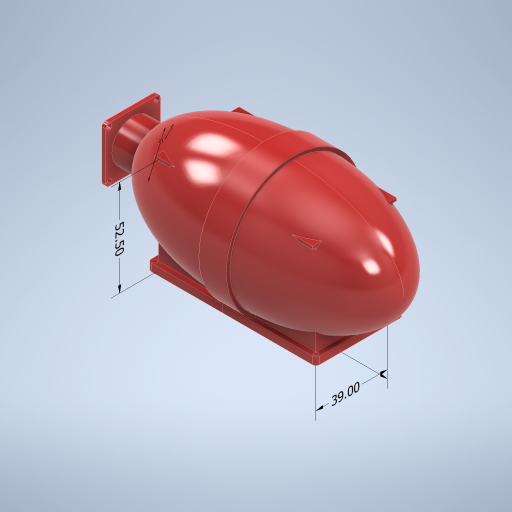
# Autodesk Inventor part: Submarino
Saved by Autodesk Inventor 2023 (Build 270158000, 158)
## iProperties
Created: 2023-03-17
Part Number: Submarino
Material: Plástico PET
Document SubType Name: Modeling
Designer: sergi
Density: 1.541 g/cm^3
Appearance: Rojo naranja
Author: sergi
Autodesk Inventor part; units mm, degrees
note: some values were not read from the file. Chosen so that the rebuilt part matches the saved one: direction of "Agujero2"; direction of "Agujero3"; direction of "Agujero4"; direction of "Agujero5"; direction of "Agujero6"; direction of "Agujero7"; direction of "Agujero8".
ref_plane "XZ Plane" through (0, 0, 0) normal (0, 1, 0) x (-1, 0, 0)
ref_plane "XY Plane" through (0, 0, 0) normal (0, 0, 1) x (1, 0, 0)
sketch "Boceto1" plane through (0, 0, 0) normal (0, 0, 1) x (1, 0, 0)
  line L0 (0, 0) -> (-65, 0)
  line L1 (0, 0) -> (0, 35)
  ellipse E0 centre (0, 0) end of major axis (-65, 0) minor radius 35
  line L2 (0, 0) -> (-63.25, 0)
  line L3 (0, 0) -> (0, 33.25)
  ellipse E1 centre (0, 0) end of major axis (-63.25, 0) minor radius 33.25
  line L4 (0, 0) -> (65, 0)
  point P0 (63.25, 0)
  dimension "d0" = 65
  dimension "d1" = 35
  dimension "d2" = 63.25
  dimension "d3" = 33.25
  constraints: 10 end point, 4 horizontal, 2 coincident, 2 point on line, 1 vertical, 9 other
  measures "d0" distance of L0.start L0.end
  measures "d1" distance of L0.start L1.end
  measures "d2" distance of L2.start L2.end
  measures "d3" distance of L2.start L3.end
revolve "Revolución1" add sketch "Boceto1" angle 360 about axis through (0, 0, 0) along (-1, 0, 0) contours L0 E0 L1 E1 | L1 E0 L4 E1
sketch "Boceto4" plane through (0, 0, 0) normal (0, 1, 0) x (-1, 0, 0)
  line L0 (-36.5, -19.5) -> (36.5, -19.5)
  line L1 (36.5, -19.5) -> (36.5, 19.5)
  line L2 (36.5, 19.5) -> (-36.5, 19.5)
  line L3 (-36.5, 19.5) -> (-36.5, -19.5)
  line L4 (-36.5, -19.5) -> (36.5, 19.5) construction
  line L5 (36.5, -19.5) -> (-36.5, 19.5) construction
  line L6 (-19.5, -14.5) -> (19.5, 14.5) construction
  line L7 (19.5, -14.5) -> (-19.5, 14.5) construction
  line L8 (-38, -21) -> (38, -21)
  line L9 (38, -21) -> (38, 21)
  line L10 (38, 21) -> (-38, 21)
  line L11 (-38, 21) -> (-38, -21)
  line L12 (-38, -21) -> (38, 21) construction
  line L13 (38, -21) -> (-38, 21) construction
  point P0 (0, 0)
  dimension "d21" = 76
  dimension "d22" = 42
  dimension "d44" = 1.5
  dimension "d45" = 1.5
  constraints: 28 end point, 6 midpoint, 4 parallel, 2 horizontal, 2 perpendicular
  measures "d21" distance of L10.end L9.end
  measures "d22" distance of L10.end L8.start
  measures "d44" distance between parallel lines of L10 L2
  measures "d45" distance between parallel lines of L9 L1
extrude "Extrusión1" add sketch "Boceto4" along normal blind 22 and the other way blind 33
extrude "Extrusión2" cut sketch "Boceto4" along normal blind 22 and the other way blind 35 contours L3 L2 L1 L0
sketch "Boceto6" plane through (0, 0, 0) normal (0, 0, 1) x (1, 0, 0)
  point P0 (0, 0)
ref_plane "Plano de trabajo1" through (-60, 0, 0) normal (1, 0, 0) x (0, 1, 0)
sketch "Boceto9" plane through (-60, 0, 0) normal (1, 0, 0) x (0, 1, 0)
  circle A0 centre (0, 0) radius 11.5
  circle A1 centre (0, 0) radius 8.5
  dimension "d46" = 23
  dimension "d49" = 3
  constraints: 2 centre point, 2 coincident
  measures "d46" diameter of A0
  measures "d49" radial gap between concentric circles of A0 A1
extrude "Extrusión5" cut sketch "Boceto9" against normal blind 30 contours A0 | A1
extrude "Extrusión7" cut sketch "Boceto9" along normal blind 10
extrude "Extrusión8" add sketch "Boceto9" along normal mid plane 30
sketch "Boceto10" plane through (-75, 0, 0) normal (-1, 0, 0) x (0, 0, 1)
  line L0 (13, -15) -> (-13, -15)
  line L1 (-15, -13) -> (-15, 13)
  line L2 (-13, 15) -> (13, 15)
  line L3 (15, 13) -> (15, -13)
  line L4 (0, 33.25) -> (0, 0) projected
  line L5 (15, -15) -> (-15, 15) construction
  line L6 (-15, -15) -> (15, 15) construction
  circle A0 centre (0, 0) radius 11.5
  arc A1 (-13, 15) -> (-15, 13) centre (-13, 13) ccw
  arc A2 (-15, -13) -> (-13, -15) centre (-13, -13) ccw
  arc A3 (13, -15) -> (15, -13) centre (13, -13) ccw
  arc A4 (15, 13) -> (13, 15) centre (13, 13) ccw
  point P0 (0, 11.5)
  dimension "d56" = 30
  dimension "d57" = 30
  dimension "d104" = 2
  constraints: 12 end point, 8 point on circle, 8 point on line, 8 tangent, 5 centre point, 3 equal radius, 2 midpoint, 2 parallel, 1 coincident, 1 horizontal, 1 perpendicular
  measures "d56" distance of L5.end L6.end
  measures "d57" distance of L6.start L5.end
  measures "d104" radius of A1
extrude "Extrusión9" add sketch "Boceto10" against normal blind 2
sketch "Boceto12" plane through (0, 22, 0) normal (0, 1, 0) x (1, 0, 0)
  line L0 (-38, 21) -> (38, -21) construction
  line L1 (35, 20) -> (-35, -20) construction
  line L2 (-38, -23) -> (38, -23)
  line L3 (38, -23) -> (38, 23)
  line L4 (38, 23) -> (-38, 23)
  line L5 (-38, 23) -> (-38, -23)
  line L6 (-38, -23) -> (38, 23) construction
  line L7 (38, -23) -> (-38, 23) construction
  point P0 (0, 0)
  dimension "d80" = 76
  dimension "d81" = 46
  constraints: 16 end point, 4 midpoint, 2 parallel, 1 horizontal, 1 perpendicular
  measures "d80" distance of L3.end L4.end
  measures "d81" distance of L4.end L2.start
extrude "Extrusión10" add sketch "Boceto12" against normal blind 1.5
sketch "Boceto14" plane through (0, -33, 0) normal (0, -1, 0) x (1, 0, 0)
  line L0 (38, 21) -> (-38, 21) projected
  line L1 (38, -21) -> (-38, -21)
  line L2 (-38, -21) -> (-38, 21)
  line L3 (-38, 21) -> (38, 21)
  line L4 (38, 21) -> (38, -21)
  line L5 (38, -21) -> (-38, 21) construction
  line L6 (-38, -21) -> (38, 21) construction
  line L7 (39, -24) -> (-39, -24)
  line L8 (-41, -22) -> (-41, 22)
  line L9 (-39, 24) -> (39, 24)
  line L10 (41, 22) -> (41, -22)
  line L11 (41, -24) -> (-41, 24) construction
  line L12 (-41, -24) -> (41, 24) construction
  arc A0 (-39, 24) -> (-41, 22) centre (-39, 22) ccw
  arc A1 (41, 22) -> (39, 24) centre (39, 22) ccw
  arc A2 (39, -24) -> (41, -22) centre (39, -22) ccw
  arc A3 (-41, -22) -> (-39, -24) centre (-39, -22) ccw
  point P0 (0, 0)
  dimension "d82" = 3
  dimension "d83" = 3
  dimension "d99" = 2
  dimension "d140" = 82
  dimension "d141" = 48
  constraints: 24 end point, 8 point on circle, 8 point on line, 8 tangent, 4 centre point, 4 midpoint, 4 parallel, 3 equal radius, 2 horizontal, 2 perpendicular
  measures "d82" distance between parallel lines of L7 L1
  measures "d83" distance between parallel lines of L10 L4
  measures "d99" radius of A0
  measures "d140" distance between parallel lines of L8 L10
  measures "d141" distance between parallel lines of L9 L7
extrude "Extrusión11" add sketch "Boceto14" against normal blind 4
sketch "Boceto13" plane through (0, 0, 0) normal (0, 0, 1) x (1, 0, 0)
  point P0 (0, 0)
sketch "Boceto16" plane through (0, -33, 0) normal (0, -1, 0) x (1, 0, 0)
  line L0 (-36.5, 19.5) -> (36.5, 19.5) projected
  line L1 (36.5, -19.5) -> (-36.5, -19.5)
  line L2 (-36.5, -19.5) -> (-36.5, 19.5)
  line L3 (-36.5, 19.5) -> (36.5, 19.5)
  line L4 (36.5, 19.5) -> (36.5, -19.5)
  line L5 (36.5, -19.5) -> (-36.5, 19.5) construction
  line L6 (-36.5, -19.5) -> (36.5, 19.5) construction
  line L7 (-38, -21) -> (38, -21)
  line L8 (38, -21) -> (38, 21)
  line L9 (38, 21) -> (-38, 21)
  line L10 (-38, 21) -> (-38, -21)
  line L11 (-38, -21) -> (38, 21) construction
  line L12 (38, -21) -> (-38, 21) construction
  point P0 (0, 0)
  dimension "d100" = 1.5
  dimension "d101" = 1.5
  constraints: 24 end point, 4 midpoint, 4 parallel, 2 horizontal, 2 perpendicular
  measures "d100" distance between parallel lines of L8 L4
  measures "d101" distance between parallel lines of L9 L0
extrude "Extrusión13" cut sketch "Boceto16" against normal blind 1
sketch "Boceto17" plane through (-75, 0, 0) normal (-1, 0, 0) x (0, 0, 1)
  line L0 (10, -10) -> (-10, -10)
  line L1 (-10, -10) -> (-10, 10)
  line L2 (-10, 10) -> (10, 10)
  line L3 (10, 10) -> (10, -10)
  line L4 (0, 33.25) -> (0, 0) projected
  line L5 (10, -10) -> (-10, 10) construction
  line L6 (-10, -10) -> (10, 10) construction
  line L7 (11, -11) -> (-11, -11)
  line L8 (-11, -11) -> (-11, 11)
  line L9 (-11, 11) -> (11, 11)
  line L10 (11, 11) -> (11, -11)
  line L11 (11, -11) -> (-11, 11) construction
  line L12 (-11, -11) -> (11, 11) construction
  point P0 (0, 11.5)
  dimension "d105" = 1
  dimension "d106" = 1
  dimension "d107" = 10
  constraints: 24 end point, 4 midpoint, 4 parallel, 2 horizontal, 2 perpendicular, 1 point on line
  measures "d105" distance between parallel lines of L9 L2
  measures "d106" distance between parallel lines of L10 L3
  measures "d107" distance from line of L4.end L3
extrude "Extrusión14" cut sketch "Boceto17" against normal blind 1
sketch "Boceto19" plane through (-73, 0, 0) normal (1, 0, 0) x (0, 0, -1)
  point P0 (13, -13)
  point P1 (13, 13)
hole "Agujero2" at (-73, -13, -13) at (-73, 13, -13) direction (-1, 0, 0) diameter 2.9 depth 2
sketch "Boceto20" plane through (-73, 0, 0) normal (1, 0, 0) x (0, 0, -1)
  point P0 (-13, 13)
hole "Agujero3" at (-73, 13, 13) direction (-1, 0, 0) diameter 2.9 depth 2
sketch "Boceto21" plane through (-73, 0, 0) normal (1, 0, 0) x (0, 0, -1)
  point P0 (-13, -13)
hole "Agujero4" at (-73, -13, 13) direction (-1, 0, 0) diameter 2.9 depth 2
sketch "Boceto22" plane through (0, -29, 0) normal (0, 1, 0) x (1, 0, 0)
  point P0 (39, 22)
hole "Agujero5" at (39, -29, -22) direction (0, -1, 0) diameter 2.4 depth 4
sketch "Boceto23" plane through (0, -29, 0) normal (0, 1, 0) x (1, 0, 0)
  point P0 (39, -22)
hole "Agujero6" at (39, -29, 22) direction (0, -1, 0) diameter 2.4 depth 4
sketch "Boceto24" plane through (0, -29, 0) normal (0, 1, 0) x (1, 0, 0)
  point P0 (-39, 22)
hole "Agujero7" at (-39, -29, -22) direction (0, -1, 0) diameter 2.4 depth 4
sketch "Boceto25" plane through (0, -29, 0) normal (0, 1, 0) x (1, 0, 0)
  point P0 (-39, -22)
hole "Agujero8" at (-39, -29, 22) direction (0, -1, 0) diameter 2.4 depth 4
sketch "Sketch26" plane through (0, 0, 0) normal (0, 0, 1) x (1, 0, 0)
  point P0 (0, 0)
split body "Split1" result two bodies by plane through (0, 0, 0) normal (1, 0, 0) first body at (8.7367, -20.0077, -27.7135)
move or copy body "Move2" bodies to move or copy 2 copy no translate (10, 0, 0)
sketch "Sketch27" plane through (0, -32, 19.5) normal (1, 0, 0) x (0, 0, -1)
  arc A0 (39, 2.9354) -> (0, 2.9354) centre (19.5, 32) ccw
  line L0 (-1.5, 3) -> (-1.5, 12.8865) projected
  line L1 (-2.5, 3) -> (-4.5, 3) projected
  line L2 (-1.5, 3) -> (-4.5, 3)
  line L3 (-4.5, -1) -> (-4.5, 3) projected
  line L4 (-4.5, 3) -> (-4.5, -1)
  line L5 (-4.5, -1) -> (-1.5, -1)
  line L6 (40.5, 0) -> (-1.5, 0) projected
  line L7 (-1.5, -1) -> (-1.5, 0)
  line L8 (0, 52.5) -> (0, 0) projected
  line L9 (-1.5, 0) -> (0, 0)
  line L10 (39, 0) -> (39, 52.5) projected
  line L11 (39, 2.9354) -> (39, 0)
  line L12 (40.5, -1) -> (40.5, 0) projected
  line L13 (39, 0) -> (40.5, 0)
  line L14 (40.5, 0) -> (40.5, -1)
  line L15 (43.5, -1) -> (43.5, 3) projected
  line L16 (40.5, -1) -> (43.5, -1)
  line L17 (43.5, 3) -> (41.5, 3) projected
  line L18 (43.5, -1) -> (43.5, 3)
  line L19 (40.5, 12.8865) -> (40.5, 3) projected
  line L20 (43.5, 3) -> (40.5, 3)
  line L21 (40.5, 3) -> (40.5, 4)
  line L22 (39, 2.9354) -> (39, 5.0684)
  line L23 (0, 2.9354) -> (0, 5.0684)
  line L24 (-1.5, 51.1135) -> (-1.5, 52.5) projected
  line L25 (-1.5, 6.2209) -> (-1.5, 52.5)
  line L26 (-3.5, 52.5) -> (-1.5, 52.5) projected
  line L27 (-1.5, 52.5) -> (-3.5, 52.5)
  line L28 (-3.5, 54) -> (42.5, 54) projected
  line L29 (-3.5, 52.5) -> (-3.5, 54)
  line L30 (-3.5, 54) -> (42.5, 54)
  line L31 (42.5, 52.5) -> (40.5, 52.5) projected
  line L32 (42.5, 54) -> (42.5, 52.5)
  line L33 (42.5, 52.5) -> (40.5, 52.5)
  line L34 (40.5, 52.5) -> (40.5, 6.2209)
  line L35 (39, 52.5) -> (0, 52.5) projected
  line L36 (39, 52.5) -> (39, 5.0684)
  line L37 (39, 52.5) -> (0, 52.5)
  line L38 (0, 52.5) -> (0, 5.0684)
  arc A1 (0, 5.0684) -> (10.4688, 0) centre (19.5, 32) ccw
  arc A2 (40.5, 6.2209) -> (-1.5, 6.2209) centre (19.5, 32) ccw
  dimension "d185" = 70
  constraints: 48 end point, 12 perpendicular, 8 point on line, 7 point on circle, 4 collinear, 3 centre point, 2 coincident, 1 horizontal, 1 parallel, 1 vertical
  measures "d185" diameter of A0
extrude "Extrusion15" add sketch "Sketch27" along normal blind 10 contours L10 L35 L8 A0 L0 L25 L24 L26 L29 L28 L32 L31 L34 L19 | L19 A2 L0 A0 bodies 3
sketch "Sketch28" plane through (10, -32, -19.5) normal (-1, 0, 0) x (0, 0, 1)
  line L0 (19.5, 65.25) -> (19.5, 32) projected
  arc A0 (39, 2.9354) -> (0, 2.9354) centre (19.5, 32) ccw
  arc A1 (42.4783, 3) -> (-3.4783, 3) centre (19.5, 32) ccw
  line L1 (-3.7, 3) -> (-1.3, 3) projected
  line L2 (-3.4783, 3) -> (-4.5, 3)
  line L3 (-4.5, 3) -> (-4.5, -1) projected
  line L4 (-4.5, 3) -> (-4.5, -1)
  line L5 (-4.5, -1) -> (-1.5, -1) projected
  line L6 (-4.5, -1) -> (-1.5, -1)
  line L7 (-1.5, -1) -> (-1.5, 0)
  line L8 (0, 52.5) -> (0, 0) projected
  line L9 (-1.5, 0) -> (0, 0)
  line L10 (0, 0) -> (0, 0.5556)
  line L11 (0, 2.9354) -> (0, 0.5556)
  line L12 (39, 0) -> (39, 52.5) projected
  line L13 (39, 2.9354) -> (39, 0)
  line L14 (40.5, 0) -> (-1.5, 0) projected
  line L15 (40.5, -1) -> (40.5, 0) projected
  line L16 (39, 0) -> (40.5, 0)
  line L17 (40.5, 0) -> (40.5, -1)
  line L18 (40.5, -1) -> (43.5, -1) projected
  line L19 (40.5, -1) -> (43.5, -1)
  line L20 (43.5, 3) -> (40.5, 3) projected
  line L21 (43.5, -1) -> (43.5, 3)
  line L22 (40.5, 3) -> (40.5, 12.8865) projected
  line L23 (43.5, 3) -> (42.4783, 3)
  point P0 (42.4783, 3)
  point P1 (-4.5, 3)
  dimension "d189" = 70
  dimension "d190" = 74
  constraints: 26 end point, 7 perpendicular, 5 point on line, 4 point on circle, 3 collinear, 2 centre point, 2 coincident, 1 horizontal, 1 vertical
  measures "d189" diameter of A0
  measures "d190" diameter of A1
extrude "Extrusion16" add sketch "Sketch28" along normal blind 10 and the other way blind 5 contours A0 L22 L20 L21 L18 L15 L14 L12 | A0 L8 L9 L7 L5 L3 L2 L1 A1 L20 L22 bodies 2
body "Solid2"
body "Solid3"
